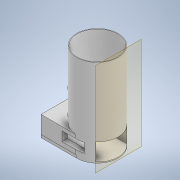
# Autodesk Inventor part: HousingMKIII
Saved by Autodesk Inventor 2021 (Build 250183000, 183)
## iProperties
Created: 2020-06-27
Part Number: HousingMKIII
Material: Generic
Document SubType Name: Modeling
Designer: Jaysonn
Density: 1 g/cm^3
Appearance: Default
Author: Jaysonn
## iProperties of the stored document _3DPrint.ipt
Created: 2020-06-27
Part Number: _3DPrint
Material: Generic
Document SubType Name: Modeling
Designer: Jaysonn
Density: 1 g/cm^3
Appearance: Default
Author: Jaysonn
Autodesk Inventor part; units mm, degrees
ref_plane "XZ Plane" through (0, 0, 0) normal (0, 1, 0) x (-1, 0, 0)
ref_plane "XY Plane" through (0, 0, 0) normal (0, 0, 1) x (1, 0, 0)
sketch "Sketch1" plane through (0, 0, 0) normal (0, 1, 0) x (-1, 0, 0)
  circle A0 centre (0, 0) radius 39.37
  dimension "d0" = 78.74
  constraints: 1 centre point, 1 coincident
  measures "d0" diameter of A0
extrude "Extrusion1" add sketch "Sketch1" along normal blind 127
sketch "Sketch2" plane through (0, 127, 0) normal (0, 1, 0) x (1, 0, 0)
  circle A0 centre (0, 0) radius 38.1
  dimension "d3" = 76.2
  constraints: 1 centre point, 1 coincident
  measures "d3" diameter of A0
extrude "Extrusion2" cut sketch "Sketch2" against normal blind 127
sketch "Sketch3" plane through (0, 0, 0) normal (0, -1, 0) x (1, 0, 0)
  circle A0 centre (0, 0) radius 39.37
  constraints: 1 centre point, 1 coincident
extrude "Extrusion3" add sketch "Sketch3" along normal blind 33.02
sketch "Sketch4" plane through (0, 0, 0) normal (1, 0, 0) x (0, 1, 0)
  line L0 (-33.02, 39.37) -> (-33.02, -39.37) projected
  line L1 (0, 39.2884) -> (-33.02, 39.2884)
  line L2 (-33.02, 39.2884) -> (-33.02, -39.37)
  line L3 (-33.02, -39.37) -> (0, -39.37)
  line L4 (0, -39.37) -> (0, 39.2884)
  point P0 (0, 0)
  constraints: 8 end point, 2 parallel, 1 horizontal, 1 perpendicular
extrude "Extrusion4" add sketch "Sketch4" against normal blind 67.31
ref_plane "Work Plane1" through (39.37, 0, 0) normal (1, 0, 0) x (0, 1, 0)
sketch "Sketch5" plane through (39.37, 0, 0) normal (1, 0, 0) x (0, 1, 0)
  line L0 (-3.1755, 0) -> (-31.1155, 0)
  line L1 (-31.1155, 0) -> (-31.1155, 29.21)
  line L2 (-31.1155, 29.21) -> (-3.1755, 29.21)
  line L3 (-3.1755, 29.21) -> (-3.1755, 0)
  line L4 (-3.1755, 0) -> (-31.1155, 0)
  line L5 (-31.1155, 0) -> (-31.1155, -29.845)
  line L6 (-31.1155, -29.845) -> (-3.1755, -29.845)
  line L7 (-3.1755, -29.845) -> (-3.1755, 0)
  point P0 (0, 0)
  dimension "d10" = 27.94
  dimension "d11" = 29.21
  dimension "d12" = 27.94
  dimension "d13" = 29.845
  constraints: 16 end point, 4 parallel, 2 horizontal, 2 perpendicular
  measures "d10" distance of L1.end L2.end
  measures "d11" distance of L0.end L1.end
  measures "d12" distance of L6.end L5.end
  measures "d13" distance of L5.end L4.end
extrude "Extrusion5" cut sketch "Sketch5" against normal blind 103.8225
sketch "Sketch6" plane through (0, 0, 0) normal (0, 0, 1) x (1, 0, 0)
  line L0 (39.37, -33.02) -> (39.37, 127) projected
  line L1 (39.37, -2.744) -> (13.0341, -2.744)
  line L2 (13.0341, -2.744) -> (-104.9586, 63.1124)
  line L3 (13.0341, -6.86) -> (-27.6059, -6.86)
  line L4 (-27.6059, -6.86) -> (-27.6059, -24.64)
  line L5 (-27.6059, -24.64) -> (13.0341, -24.64)
  line L6 (13.0341, -24.64) -> (13.0341, -6.86)
  point P0 (0, 0)
  dimension "d16" = 40.64
  dimension "d17" = 17.78
  constraints: 12 end point, 2 horizontal, 2 parallel, 1 perpendicular, 1 point on line
  measures "d16" distance of L5.end L4.end
  measures "d17" distance of L4.end L3.end
extrude "Extrusion6" cut sketch "Sketch6" along normal blind 102.5525
sketch "Sketch7" plane through (0, 0, 0) normal (0, 0, 1) x (1, 0, 0)
  point P0 (0, 0)
sketch "Sketch8" plane through (0, 0, 0) normal (0, 0, 1) x (1, 0, 0)
  point P0 (0, 0)
sketch "Sketch9" plane through (0, 0, 0) normal (0, 0, 1) x (1, 0, 0)
  point P0 (0, 0)
sketch "Sketch10" plane through (0, 0, 0) normal (0, 0, 1) x (1, 0, 0)
  line L0 (0, 7.3743) -> (-17.78, 7.3743)
  line L1 (-17.78, 7.3743) -> (-17.78, 30.2343)
  line L2 (-17.78, 30.2343) -> (0, 30.2343)
  line L3 (0, 30.2343) -> (0, 7.3743)
  point P0 (0, 0)
  dimension "d20" = 17.78
  dimension "d21" = 22.86
  constraints: 8 end point, 2 parallel, 1 horizontal, 1 perpendicular
  measures "d20" distance of L1.end L2.end
  measures "d21" distance of L0.end L1.end
extrude "Extrusion7" cut sketch "Sketch10" against normal blind 102.5525
sketch "Sketch11" plane through (0, 0, 0) normal (1, 0, 0) x (0, 1, 0)
  line L0 (127, -39.37) -> (127, 39.37) projected
  line L1 (127, 0) -> (68.58, 0)
  line L2 (68.58, 0) -> (68.58, 25.4)
  line L3 (59.5338, 0) -> (59.5338, -25.4)
  line L4 (59.5338, -25.4) -> (54.4538, -25.4)
  line L5 (54.4538, -25.4) -> (54.4538, -27.94)
  line L6 (54.4538, -27.94) -> (59.5338, -27.94)
  line L7 (59.5338, -27.94) -> (59.5338, -25.4)
  line L8 (59.5338, 25.4) -> (54.4538, 25.4)
  line L9 (54.4538, 25.4) -> (54.4538, 27.94)
  line L10 (54.4538, 27.94) -> (59.5338, 27.94)
  line L11 (59.5338, 27.94) -> (59.5338, 25.4)
  line L12 (15.2971, -27.94) -> (10.2171, -27.94)
  line L13 (10.2171, -27.94) -> (10.2171, -25.4)
  line L14 (10.2171, -25.4) -> (15.2971, -25.4)
  line L15 (15.2971, -25.4) -> (15.2971, -27.94)
  line L16 (15.2971, 25.4) -> (10.2171, 25.4)
  line L17 (10.2171, 25.4) -> (10.2171, 27.94)
  line L18 (10.2171, 27.94) -> (15.2971, 27.94)
  line L19 (15.2971, 27.94) -> (15.2971, 25.4)
  point P0 (0, 0)
  dimension "d24" = 58.42
  dimension "d25" = 25.4
  dimension "d26" = 25.4
  dimension "d27" = 5.08
  dimension "d28" = 2.54
  dimension "d29" = 5.08
  dimension "d30" = 2.54
  dimension "d31" = 5.08
  dimension "d32" = 2.54
  constraints: 38 end point, 8 parallel, 6 point on line, 5 horizontal, 4 perpendicular, 2 vertical, 1 midpoint
  measures "d24" distance of L1.start L1.end
  measures "d25" distance of L1.end L2.end
  measures "d26" distance of L3.start L3.end
  measures "d27" distance of L6.end L5.end
  measures "d28" distance of L5.end L4.end
  measures "d29" distance of L9.end L10.end
  measures "d30" distance of L8.end L9.end
  measures "d31" distance of L13.end L14.end
  measures "d32" distance of L12.end L13.end
extrude "Extrusion8" cut sketch "Sketch11" against normal blind 83.185
sketch "Sketch12" plane through (0, -33.02, 0) normal (0, -1, 0) x (1, 0, 0)
  point P0 (0, 0)
sketch "Sketch13" plane through (0, -33.02, 0) normal (0, -1, 0) x (1, 0, 0)
  circle A0 centre (0, 0) radius 39.37
  dimension "d35" = 78.74
  constraints: 1 centre point, 1 coincident
  measures "d35" diameter of A0
extrude "Extrusion9" add sketch "Sketch13" along normal blind 5.08
sketch "Sketch14" plane through (0, -33.02, 0) normal (0, -1, 0) x (1, 0, 0)
  circle A0 centre (0, 0) radius 39.37 projected
  line L0 (0, -39.37) -> (-67.31, -39.37) projected
  line L1 (0, 39.37) -> (-67.31, 39.37)
  line L2 (-67.31, 39.37) -> (-67.31, -39.37)
  line L3 (-67.31, -39.37) -> (0, -39.37)
  line L4 (0, -39.37) -> (0, 39.37)
  constraints: 8 end point, 2 parallel, 1 horizontal, 1 perpendicular, 1 point on circle
extrude "Extrusion10" add sketch "Sketch14" along normal blind 5.08 contours A0 L0 L2 L1
sketch "Sketch15" plane through (39.37, 0, 0) normal (1, 0, 0) x (0, 1, 0)
  line L0 (-31.1155, 29.21) -> (-31.1155, -29.845) projected
  line L1 (-31.1155, 29.21) -> (-36.1955, 29.21)
  line L2 (-36.1955, 29.21) -> (-36.1955, -29.845)
  line L3 (-36.1955, -29.845) -> (-31.1155, -29.845)
  line L4 (-31.1155, -29.845) -> (-31.1155, 29.21)
  point P0 (0, 0)
  dimension "d40" = 5.08
  dimension "d41" = 59.055
  constraints: 8 end point, 2 parallel, 1 horizontal, 1 perpendicular
  measures "d40" distance of L3.end L2.end
  measures "d41" distance of L2.end L1.end
extrude "Extrusion11" cut sketch "Sketch15" against normal blind 104.14
body "Solid1"
